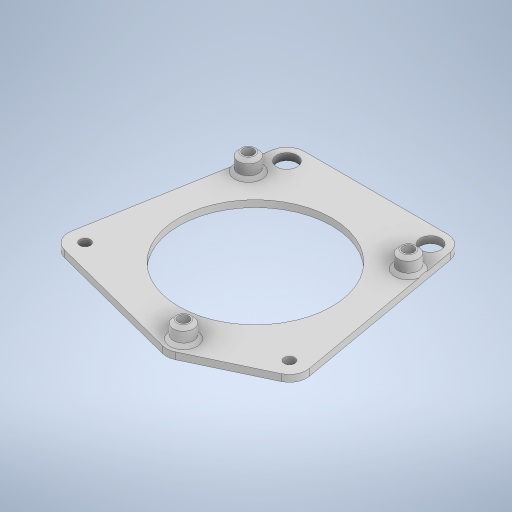
# Autodesk Inventor part: SimpleRTK - PlateAdapter
Saved by Autodesk Inventor 2023 (Build 270158000, 158)
## iProperties
Created: 2023-01-25
Part Number: SimpleRTK - PlateAdapter
Material: Generic
Document SubType Name: Modeling
Designer: Administrator
Density: 1 g/cm^3
Appearance: Default
Author: Administrator
Autodesk Inventor part; units mm, degrees
ref_plane "YZ Plane" through (0, 0, 0) normal (1, 0, 0) x (0, 1, 0)
ref_plane "XZ Plane" through (0, 0, 0) normal (0, 1, 0) x (-1, 0, 0)
ref_plane "XY Plane" through (0, 0, 0) normal (0, 0, 1) x (1, 0, 0)
sketch "Sketch1" plane through (0, 0, 0) normal (0, 0, 1) x (1, 0, 0)
  circle A0 centre (8.9, 50.3645) radius 1.55 construction
  circle A1 centre (8.9, 50.3645) radius 3
  circle A2 centre (51.1, 50.3645) radius 1.55 construction
  circle A3 centre (51.1, 50.3645) radius 3
  circle A4 centre (60, 0) radius 1.55
  circle A5 centre (60, 0) radius 1.55
  circle A6 centre (0, 0) radius 1.55
  circle A7 centre (0, 0) radius 1.55
  circle A8 centre (54.13, 40.8) radius 1.5999
  circle A9 centre (5.87, 42.07) radius 1.5999
  circle A10 centre (38.89, -10) radius 1.5999
  circle A11 centre (54.13, 40.8) radius 1.55 construction
  circle A12 centre (5.87, 42.07) radius 1.55 construction
  circle A13 centre (38.89, -10) radius 1.55 construction
  line L0 (8.9, 55.3645) -> (3.9, 55.3645) construction
  circle A14 centre (30, 20) radius 22.5
  arc A15 (38.89, -5) -> (37.7654, -14.8719) centre (38.89, -10) ccw construction
  arc A16 (37.6448, -14.8425) -> (41.0305, -14.5186) centre (38.89, -10) ccw
  line L1 (8.9, 55.3645) -> (8.9, 50.3645) construction
  line L2 (51.1, 55.3645) -> (51.1, 50.3645) construction
  arc A17 (-1.2452, -4.8425) -> (-5, 0) centre (0, 0) ccw construction
  arc A18 (65, 0) -> (64.9237, 0.8701) centre (60, 0) ccw
  line L3 (-1.2452, -4.8425) -> (37.6448, -14.8425)
  line L4 (41.0305, -14.5186) -> (62.1405, -4.5186)
  arc A19 (-4.9237, 0.8701) -> (-1.2452, -4.8425) centre (0, 0) ccw
  arc A20 (62.1405, -4.5186) -> (65, 0) centre (60, 0) ccw
  arc A21 (3.9763, 51.2346) -> (8.9, 55.3645) centre (8.9, 50.3645) ccw construction
  line L5 (-4.9237, 0.8701) -> (3.9763, 51.2346)
  line L6 (56.0237, 51.2346) -> (64.9237, 0.8701)
  arc A22 (64.9237, 0.8701) -> (62.1405, -4.5186) centre (60, 0) ccw construction
  arc A23 (41.0305, -14.5186) -> (38.89, -5) centre (38.89, -10) ccw construction
  line L7 (8.9, 55.3645) -> (51.1, 55.3645)
  arc A24 (8.9, 55.3645) -> (3.9763, 51.2346) centre (8.9, 50.3645) ccw
  circle A25 centre (51.1, 50.3645) radius 5
  point P0 (17, 90.5)
  dimension "d0" = 6
  dimension "d1" = 6
  dimension "d2" = 3.1
  dimension "d3" = 3.1
  dimension "d4" = 8.9
  dimension "d5" = 8.9
  dimension "d6" = 42.2
  dimension "d7" = 50.3645
  dimension "d8" = 0
  dimension "d9" = 0
  dimension "d10" = 3.1
  dimension "d11" = 3.1
  dimension "d12" = 3.1
  dimension "d13" = 52.07
  dimension "d14" = 50.8
  dimension "d15" = 33.02
  dimension "d16" = 15.24
  dimension "d19" = 5.87
  dimension "d51" = 5
  dimension "d52" = 45
  dimension "d55" = 10
  dimension "d56" = 10
  dimension "d65" = 20
  dimension "d66" = 21.1
  dimension "d67" = 10
  dimension "d68" = 10
  dimension "d69" = 10
  dimension "d71" = 10
  constraints: 26 centre point, 23 point on circle, 16 end point, 12 coincident, 11 tangent, 2 vertical, 1 horizontal
  measures "d0" diameter of A1
  measures "d1" diameter of A3
  measures "d2" diameter of A5
  measures "d3" diameter of A7
  measures "d4" horizontal distance of point (0, 0) A1.centre
  measures "d5" horizontal distance of A5.centre A3.centre
  measures "d6" distance of A3.centre A1.centre
  measures "d7" vertical distance of point (0, 0) A1.centre
  measures "d8" vertical distance of point (0, 0) A5.centre
  measures "d9" vertical distance of A1.centre A3.centre
  measures "d10" diameter of A11
  measures "d11" diameter of A12
  measures "d12" diameter of A13
  measures "d13" vertical distance of A10.centre A9.centre
  measures "d14" vertical distance of A8.centre A10.centre
  measures "d15" horizontal distance of A10.centre A9.centre
  measures "d16" horizontal distance of A11.centre A10.centre
  measures "d19" horizontal distance of point (0, 0) A9.centre
  measures "d51" distance of L0.start L0.end
  measures "d52" diameter of A14
  measures "d55" vertical distance of A5.centre A13.centre
  measures "d56" diameter of A15
  measures "d65" vertical distance of A5.centre A14.centre
  measures "d66" horizontal distance of A3.centre A14.centre
  measures "d67" diameter of A18
  measures "d68" diameter of A17
  measures "d69" diameter of A21
  measures "d71" diameter of A25
extrude "Extrusion1" add sketch "Sketch1" along normal blind 2
sketch "Sketch5" plane through (0, 0, 2) normal (0, 0, 1) x (1, 0, 0)
  circle A0 centre (5.87, 42.07) radius 1.5999 projected
  circle A1 centre (5.87, 42.07) radius 3
  circle A2 centre (54.13, 40.8) radius 1.5999 projected
  circle A3 centre (54.13, 40.8) radius 3
  circle A4 centre (38.89, -10) radius 1.5999 projected
  circle A5 centre (38.89, -10) radius 3
  point P0 (0, 0)
  dimension "d57" = 6
  dimension "d58" = 6
  dimension "d59" = 6
  constraints: 3 centre point, 3 coincident
  measures "d57" diameter of A1
  measures "d58" diameter of A3
  measures "d59" diameter of A5
extrude "Extrusion5" add sketch "Sketch5" along normal blind 5
chamfer "Chamfer3" distance 1 angle 45 6 edges at (2.87, 42.07, 2) (2.87, 42.07, 7) (51.13, 40.8, 2) (51.13, 40.8, 7) (35.89, -10, 2) (35.89, -10, 7)
equation "\"d19\" = -0.5 * d16 - 0.5 * d15 + 0.5 * d6 + 0.5 * d5 + 0.5 * d4"
equation "\"d66\" = 0.5 * d6"
body "Solid1"
